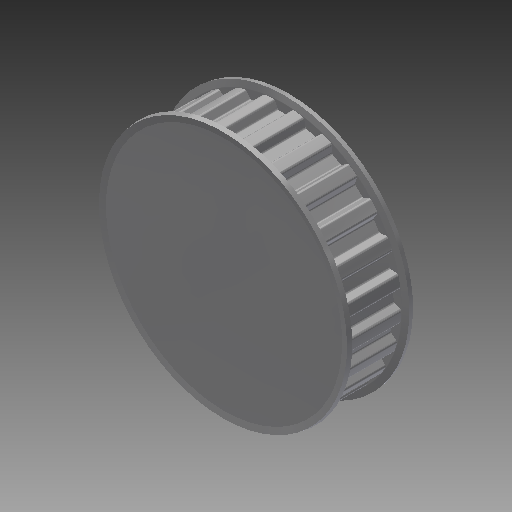
# Autodesk Inventor part: Polia síncrona2
Saved by Autodesk Inventor 2018 (Build 220112000, 112)
## iProperties
Created: 2018-09-22
Part Number: Polia síncrona2
Material: Steel
Document SubType Name: Modeling
Designer: Usuario
Density: 1 g/cm^3
Appearance: Steel
CustomPartVersion: 1
Author: Usuario
Autodesk Inventor part; units mm, degrees
ref_plane "YZ Plane" through (0, 0, 0) normal (1, 0, 0) x (0, 1, 0)
ref_plane "XZ Plane" through (0, 0, 0) normal (0, 1, 0) x (-1, 0, 0)
ref_plane "XY Plane" through (0, 0, 0) normal (0, 0, 1) x (1, 0, 0)
sketch "Esboço de polia" plane through (0, 0, 0) normal (0, 0, 1) x (1, 0, 0)
  circle A0 centre (0, 0) radius 39.7887 construction
  circle A1 centre (0, 0) radius 38.7887
  circle A2 centre (0, 0) radius 36.1887
  line L0 (-2.9597, 38.6757) -> (-1.8, 36.1887)
  line L1 (-1.8, 36.1887) -> (1.8, 36.1887)
  line L2 (1.8, 36.1887) -> (2.9597, 38.6757)
  line L3 (0, 0) -> (0, 38.7887) construction
  point P0 (0, 36.1887)
  dimension "d0" = 79.5775
  dimension "d1" = 1
  dimension "d2" = 2.6
  dimension "d3" = 50
  dimension "d4" = 3.6
  constraints: 8 end point, 3 coincident, 3 point on circle, 2 centre point, 1 horizontal, 1 midpoint, 1 point on line, 1 vertical, 1 vertical alignment, 3 other
  measures "d0" diameter of A0
  measures "d1" radial gap between concentric circles of A0 A1
  measures "d3" angle of L2 L0
  measures "d4" distance of L0.end L1.end
extrude "Corpo de base" add sketch "Esboço de polia" along normal mid plane 18 contours A2 | A1 L0 L1 L2 | L2 L1 L0 A1
extrude "Dente" cut sketch "Esboço de polia" along normal through all both and the other way through all contours L2 L1 L0 A1 picked at (0, 37.9137)
fillet "Fillet" radius 0.6 2 edges at (1.8, 36.1887, 0) (-1.8, 36.1887, 0)
fillet "Fillet" radius 0.8 4 edges at (-2.9597, 38.6757, 4.5) (-2.9597, 38.6757, -4.5) (2.9597, 38.6757, 4.5) (2.9597, 38.6757, -4.5)
pattern_circular "Dentes" count 25 over 360 about axis through (0, 0, -10) along (0, 0, 1) of "Dente", "Fillet"
pulley flange "Flange esquerdo" diameter 77.5775 height 2.2 thickness 1.5 bend angle 10 centre (0, 0, -9) toward (0, 0, -1)
pulley flange "Flange direito" diameter 77.5775 height 2.2 thickness 1.5 bend angle 10 centre (0, 0, 9) toward (0, 0, 1)
equation "\"d1\" = da_a"
equation "\"d2\" = da_hg"
equation "\"d3\" = 2 * da_fi"
equation "\"d4\" = da_bw"
equation "\"d5\" = da_bf"
equation "\"d7\" = da_bf"
equation "\"d9\" = da_rb"
equation "\"d10\" = da_rt"
equation "\"da_fi\" = 25deg"
equation "\"da_hg\" = 2.6"
equation "\"da_bw\" = 3.6"
equation "\"da_rb\" = 0.6"
equation "\"da_rt\" = 0.8"
equation "\"da_a\" = 1"
equation "\"da_bf\" = 18"
equation "\"da_wf\" = 1.5"
equation "\"da_hf\" = 2.2"
body "Solid1"
